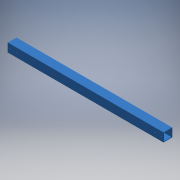
# Autodesk Inventor part: Cross Brace
Saved by Autodesk Inventor 2017 (Build 210142000, 142)
## iProperties
Created: 2017-01-15
Part Number: Cross Brace
Material: Generic
Document SubType Name: Modeling
Designer: Ben
Density: 1 g/cm^3
Appearance: Cyan
Author: Ben
Autodesk Inventor part; units mm, degrees
ref_plane "YZ Plane" through (0, 0, 0) normal (1, 0, 0) x (0, 1, 0)
ref_plane "XZ Plane" through (0, 0, 0) normal (0, 1, 0) x (-1, 0, 0)
ref_plane "XY Plane" through (0, 0, 0) normal (0, 0, 1) x (1, 0, 0)
sketch "Sketch1" plane through (0, 0, 0) normal (1, 0, 0) x (0, 1, 0)
  line L0 (11.1125, 11.1125) -> (-11.1125, 11.1125)
  line L1 (-11.1125, 11.1125) -> (-11.1125, -11.1125)
  line L2 (-11.1125, -11.1125) -> (11.1125, -11.1125)
  line L3 (11.1125, -11.1125) -> (11.1125, 11.1125)
  line L4 (12.7, 12.7) -> (-12.7, 12.7)
  line L5 (-12.7, 12.7) -> (-12.7, -12.7)
  line L6 (-12.7, -12.7) -> (12.7, -12.7)
  line L7 (12.7, -12.7) -> (12.7, 12.7)
  line L8 (0, 11.1125) -> (0, 12.7) construction
  line L9 (11.1125, 0) -> (12.7, 0) construction
  line L10 (11.1125, 0) -> (0, 0) construction
  line L11 (0, 0) -> (0, 11.1125) construction
  dimension "d0" = 25.4
  dimension "d1" = 1.5875
  constraints: 24 end point, 5 perpendicular, 4 midpoint, 4 parallel, 3 horizontal, 2 vertical
  measures "d0" distance of L4.start L4.end
  measures "d1" distance between parallel lines of L4 L0
extrude "Extrusion1" add sketch "Sketch1" along normal blind 457.2
sketch "Sketch2" plane through (0, -12.7, 12.7) normal (0, 0, 1) x (1, 0, 0)
  line L0 (0, 12.7) -> (457.2, 12.7) construction
  line L1 (457.2, 1.5875) -> (457.2, 23.8125) construction
  circle A0 centre (450.85, 12.7) radius 1.5875
  circle A1 centre (431.8, 12.7) radius 1.5875
  line L2 (228.6, 12.7) -> (228.6, 1.5875) construction
  circle A2 centre (6.35, 12.7) radius 1.5875
  circle A3 centre (25.4, 12.7) radius 1.5875
  dimension "d4" = 6.35
  dimension "d5" = 19.05
  dimension "d6" = 3.175
  constraints: 4 centre point, 4 end point, 2 midpoint, 2 point on line, 2 symmetric about line, 1 equal radius, 1 vertical, 2 other
  measures "d4" distance from line of A0.centre L1
  measures "d5" distance of A1.centre A0.centre
  measures "d6" diameter of A1
extrude "Extrusion2" cut sketch "Sketch2" against normal up to next
sketch "Sketch3" plane through (0, 12.7, 12.7) normal (0, 1, 0) x (1, 0, 0)
  line L0 (0, 0) -> (457.2, 0) construction
  line L1 (228.6, 0) -> (228.6, 42.8948) construction
  line L2 (361.95, 0) -> (361.95, 36.7793) construction
  circle A0 centre (361.95, 6.35) radius 1.5875
  circle A1 centre (361.95, 19.05) radius 1.5875
  circle A2 centre (95.25, 6.35) radius 1.5875
  circle A3 centre (95.25, 19.05) radius 1.5875
  point P0 (0, 12.7)
  dimension "d9" = 3.175
  dimension "d10" = 6.35
  dimension "d11" = 12.7
  dimension "d15" = 266.7
  constraints: 4 centre point, 4 end point, 3 point on line, 2 symmetric about line, 2 vertical, 1 equal radius, 1 midpoint, 2 other
  measures "d9" diameter of A0
  measures "d10" distance from line of L0 A0.centre
  measures "d11" distance of A0.centre A1.centre
  measures "d15" distance from line of A2.centre L2
extrude "Extrusion3" cut sketch "Sketch3" against normal up to next
body "Solid1"
